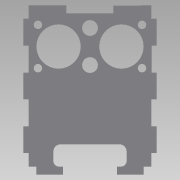
# Autodesk Inventor part: srf depan
Saved by Autodesk Inventor 2015 SP1 (Build 190203100, 203)
## iProperties
Created: 2015-02-14
Part Number: srf depan
Material: Generic
Document SubType Name: Modeling
Designer: Rafi Kurnia Putra
Density: 1 g/cm^3
Appearance: Default
Author: Rafi Kurnia Putra
Autodesk Inventor part; units mm, degrees
ref_plane "YZ Plane" through (0, 0, 0) normal (1, 0, 0) x (0, 1, 0)
ref_plane "XZ Plane" through (0, 0, 0) normal (0, 1, 0) x (-1, 0, 0)
ref_plane "XY Plane" through (0, 0, 0) normal (0, 0, 1) x (1, 0, 0)
sketch "Sketch1" plane through (0, 0, 0) normal (0, 0, 1) x (1, 0, 0)
  line L0 (23.778, 63) -> (8.751, 62.999)
  line L1 (8.7511, 59.9974) -> (8.751, 62.999)
  line L2 (-8.7484, 59.9988) -> (8.7511, 59.9974)
  line L3 (-8.7482, 62.8637) -> (-8.7484, 59.9988)
  line L4 (-8.7482, 62.8637) -> (-23.7781, 63.0002)
  circle A0 centre (11.7, 47.6838) radius 8.25
  circle A1 centre (-11.7, 47.6838) radius 8.25
  circle A2 centre (0.0002, 40.7838) radius 2.95
  circle A3 centre (19.375, 39.6228) radius 1.5875
  circle A4 centre (-19.375, 55.7448) radius 1.5875
  line L5 (10.98, 11.2972) -> (-10.98, 11.2972)
  arc A5 (13.638, 8.6392) -> (10.98, 11.2972) centre (10.98, 8.6392) ccw
  arc A6 (-10.98, 11.2972) -> (-13.638, 8.6392) centre (-10.98, 8.6392) ccw
  line L6 (-0.0001, 27) -> (-7.6501, 27) construction
  line L7 (-7.6501, 27) -> (-0.0001, 27) construction
  line L8 (-0.0001, 34) -> (-0.0001, 27) construction
  line L9 (10, 0) -> (20, 0)
  line L10 (-20, 0) -> (-10, 0)
  line L11 (-5, 0) -> (5, 0) construction
  line L12 (20, 0) -> (20, 3.0003)
  line L13 (20, 3.0003) -> (23.778, 3)
  line L14 (10, 0) -> (10, 3.0012)
  line L15 (-10, 3.0012) -> (-10, 0)
  line L16 (-20, 0) -> (-20, 3)
  line L17 (-20, 3) -> (-23.7781, 3)
  line L18 (13.638, 8.6392) -> (13.638, 5.0012)
  line L19 (-13.638, 8.6392) -> (-13.638, 5.0012)
  line L20 (11.638, 3.0012) -> (10, 3.0012)
  line L21 (-10, 3.0012) -> (-11.638, 3.0012)
  arc A7 (11.638, 3.0012) -> (13.638, 5.0012) centre (11.638, 5.0012) ccw
  arc A8 (-13.638, 5.0012) -> (-11.638, 3.0012) centre (-11.638, 5.0012) ccw
  line L22 (23.778, 28) -> (26.778, 28)
  line L23 (26.778, 28) -> (26.778, 38)
  line L24 (26.778, 38) -> (23.778, 38)
  line L25 (23.778, 48) -> (26.778, 48)
  line L26 (26.778, 48) -> (26.778, 58)
  line L27 (26.778, 58) -> (23.778, 58)
  line L28 (23.778, 8) -> (26.778, 8)
  line L29 (26.778, 8) -> (26.778, 18)
  line L30 (26.778, 18) -> (23.778, 18)
  line L31 (23.778, 28) -> (26.778, 28)
  line L32 (26.778, 28) -> (26.778, 38)
  line L33 (26.778, 38) -> (23.778, 38)
  line L34 (23.778, 48) -> (23.778, 38)
  line L35 (23.778, 28) -> (23.778, 18)
  line L36 (23.778, 8) -> (23.778, 3)
  line L37 (-23.7781, 28) -> (-26.7781, 28)
  line L38 (-26.7781, 28) -> (-26.7781, 38)
  line L39 (-26.7781, 38) -> (-23.7781, 38)
  line L40 (-26.7781, 48) -> (-26.7781, 58)
  line L41 (-26.7781, 58) -> (-23.7781, 58)
  line L42 (-23.7781, 48) -> (-26.7781, 48)
  line L43 (-26.7781, 8) -> (-26.7781, 18)
  line L44 (-26.7781, 18) -> (-23.7781, 18)
  line L45 (-23.7781, 8) -> (-26.7781, 8)
  line L46 (-26.7781, 28) -> (-26.7781, 38)
  line L47 (-26.7781, 38) -> (-23.7781, 38)
  line L48 (-23.7781, 28) -> (-26.7781, 28)
  line L49 (-23.7781, 48) -> (-23.7781, 38)
  line L50 (-23.7781, 28) -> (-23.7781, 18)
  circle A9 centre (0.0002, 54.5838) radius 2.95
  line L51 (0.0002, 50) -> (0.0002, 45) construction
  line L52 (10, 47.6838) -> (6, 47.6838) construction
  circle A10 centre (19.375, 55.7448) radius 1.5875
  circle A11 centre (-19.375, 39.6228) radius 1.5875
  line L53 (-23.7781, 3) -> (-23.7781, 8)
  line L54 (23.778, 63) -> (23.778, 58)
  line L55 (-23.7781, 63.0002) -> (-23.7781, 58)
  line L56 (23.778, 63) -> (23.778, 62.5)
  line L57 (23.778, 63) -> (22.778, 63)
  line L58 (23.778, 63) -> (24.778, 63) construction
  line L59 (22.778, 63) -> (22.778, 58)
  line L60 (22.778, 58) -> (23.778, 58)
  line L61 (23.778, 48) -> (22.778, 48)
  line L62 (22.778, 48) -> (22.778, 38)
  line L63 (22.778, 38) -> (23.778, 38)
  line L64 (23.778, 28) -> (22.778, 28)
  line L65 (22.778, 28) -> (22.778, 18)
  line L66 (22.778, 18) -> (23.778, 18)
  line L67 (23.778, 8) -> (22.778, 8)
  line L68 (22.778, 8) -> (22.7776, 3.0001)
  line L69 (-23.7781, 63.0002) -> (-23.7781, 62.5002)
  line L70 (-23.7781, 63.0002) -> (-22.7781, 62.9911)
  line L71 (-22.7781, 62.9911) -> (-22.8235, 57.9913)
  line L72 (-22.8235, 57.9913) -> (-23.7781, 58)
  line L73 (-23.7781, 48) -> (-22.9143, 47.9922)
  line L74 (-22.9143, 47.9922) -> (-23.0051, 37.9926)
  line L75 (-23.0051, 37.9926) -> (-24.0051, 38)
  line L76 (-23.7781, 28) -> (-22.7781, 28)
  line L77 (-22.7781, 28) -> (-22.7781, 18)
  line L78 (-22.7781, 18) -> (-23.7781, 18)
  line L79 (-23.7781, 8) -> (-22.7781, 8)
  line L80 (-23.7781, 8) -> (-22.7781, 8) construction
  line L81 (-22.7781, 8) -> (-22.7781, 3)
  point P0 (0, 0)
  point P1 (0, 1.5)
  point P2 (15, 0)
  point P3 (15, 1.5)
  point P4 (-15, 0)
  point P5 (-15, 1.5)
  point P6 (0, 0)
  point P7 (0, 1.5)
  point P8 (13.638, 3.0012)
  point P9 (-23.7781, 23)
  dimension "d4" = 15
  dimension "d7" = 15
  dimension "d11" = 2
  dimension "d12" = 3
  dimension "d16" = 20
  dimension "d19" = 20
  dimension "d46" = 7.675
  dimension "d47" = 7.675
  dimension "d50" = 0.5
  dimension "d51" = 1
  dimension "d52" = 180
  dimension "d53" = 10
  dimension "d54" = 10
  dimension "d55" = 90
  dimension "d56" = 1
  dimension "d57" = 0.5
  dimension "d58" = 1
  dimension "d59" = 5
  dimension "d60" = 10
  dimension "d61" = 1
  dimension "d62" = 1
  dimension "d63" = 1
  dimension "d64" = 0
  dimension "d67" = 8.061
  dimension "d68" = 8.061
  dimension "d69" = 1
  dimension "d70" = 1
  constraints: 164 end point, 18 symmetric about line, 17 vertical, 14 horizontal, 12 centre point, 12 perpendicular, 12 point on line, 8 point on circle, 5 collinear, 4 parallel, 4 tangent, 1 equal radius, 1 horizontal alignment, 1 midpoint, 39 other
  measures "d4" distance of point (0, 0) point (15, 0)
  measures "d7" distance of point (0, 0) point (-15, 0)
  measures "d11" radius of A7
  measures "d12" distance of L24.end L23.end
  measures "d16" distance of L22.end L26.start
  measures "d19" distance of L22.end L29.start
  measures "d46" horizontal distance of A4.centre A1.centre
  measures "d47" horizontal distance of A0.centre A3.centre
  measures "d50" distance of L0.start L56.end
  measures "d51" distance of L0.start L57.end
  measures "d52" angle of L57 L58
  measures "d53" distance of L61.end L62.end
  measures "d54" distance of L64.end L65.end
  measures "d55" angle of L65 L64
  measures "d56" distance of L28.start L67.end
  measures "d57" distance of L4.end L69.end
  measures "d58" distance of L4.end L70.end
  measures "d59" distance of L70.end L71.end
  measures "d60" distance of L73.end L74.end
  measures "d61" distance of L74.end L75.end
  measures "d62" distance of L48.start L76.end
  measures "d63" distance of L45.start L79.end
  measures "d64" distance between parallel lines of L79 L80
  measures "d67" vertical distance of A0.centre A3.centre
  measures "d68" vertical distance of A10.centre A0.centre
  measures "d69" distance between parallel lines of L62 L34
  measures "d70" distance between parallel lines of L65 L35
extrude "Extrusion1" add sketch "Sketch1" along normal blind 3
extrude "Extrusion2" cut sketch "Sketch1" along normal up to next contours L54 L60 L59 L0 | L34 L63 L62 L61 | L71 L72 L55 L4 | L35 L66 L65 L64 | L73 L74 L75 L49 | L36 L13 L68 L67 | L76 L77 L78 L50 | L79 L81 L17 L53
sketch "Sketch2" plane through (0, 0, 0) normal (0, 0, -1) x (-1, 0, 0)
  line L0 (-22.778, 8) -> (-26.778, 8) projected
  line L1 (-26.778, 58) -> (-24.778, 58)
  line L2 (-24.778, 58) -> (-24.778, 8)
  line L3 (-24.778, 8) -> (-26.778, 8)
  line L4 (-26.778, 8) -> (-26.778, 58)
  line L5 (26.7781, 8) -> (22.7781, 8) projected
  line L6 (26.7781, 58) -> (24.7781, 58)
  line L7 (24.7781, 58) -> (24.7781, 8)
  line L8 (24.7781, 8) -> (26.7781, 8)
  line L9 (26.7781, 8) -> (26.7781, 58)
  point P0 (0, 0)
  constraints: 16 end point, 4 parallel, 2 horizontal, 2 midpoint, 2 perpendicular
extrude "Extrusion3" cut sketch "Sketch2" against normal through all
equation "\"d56\" = d51"
equation "\"d58\" = d51"
equation "\"d61\" = d51"
equation "\"d62\" = d51"
equation "\"d63\" = d51"
equation "\"d68\" = d67"
equation "\"d69\" = d51"
equation "\"d70\" = d51"
body "Solid1"
